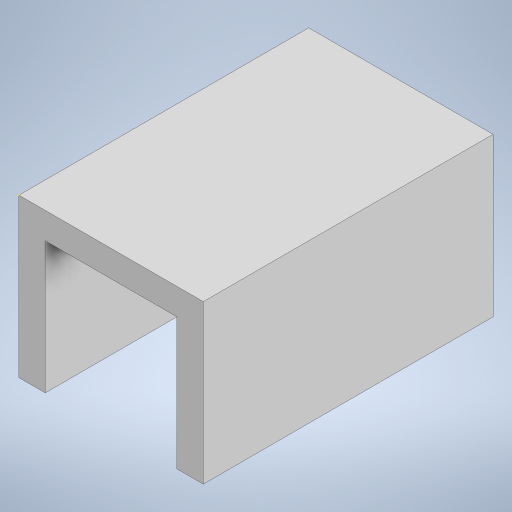
# Autodesk Inventor part: housing_v04
Saved by Autodesk Inventor 2023 (Build 270158000, 158)
## iProperties
Created: 2023-11-20
Part Number: housing_v04
Material: Generic
Document SubType Name: Modeling
Designer: Akramilab
Density: 1 g/cm^3
Appearance: Default
Author: Akramilab
Autodesk Inventor part; units mm, degrees
ref_plane "YZ Plane" through (0, 0, 0) normal (1, 0, 0) x (0, 1, 0)
ref_plane "XZ Plane" through (0, 0, 0) normal (0, 1, 0) x (-1, 0, 0)
ref_plane "XY Plane" through (0, 0, 0) normal (0, 0, 1) x (1, 0, 0)
sketch "Sketch1" plane through (0, 0, 0) normal (0, 0, 1) x (1, 0, 0)
  line L0 (0, 0) -> (14, 0)
  line L1 (14, 0) -> (14, -12)
  line L2 (14, -12) -> (0, -12)
  line L3 (0, -12) -> (0, 0)
  dimension "d0" = 14
  dimension "d1" = 12
  constraints: 8 end point, 2 parallel, 1 horizontal, 1 perpendicular
  measures "d0" distance of L1.end L2.end
  measures "d1" distance of L0.end L1.end
extrude "Extrusion1" add sketch "Sketch1" against normal blind 22
sketch "Sketch2" plane through (0, 0, 0) normal (0, 0, 1) x (1, 0, 0)
  line L0 (2, -2) -> (12, -2)
  line L1 (12, -2) -> (12, -22)
  line L2 (12, -22) -> (2, -22)
  line L3 (2, -22) -> (2, -2)
  point P0 (0, 0)
  dimension "d4" = 10
  dimension "d5" = 20
  constraints: 8 end point, 2 parallel, 1 horizontal, 1 perpendicular
  measures "d4" distance of L1.end L2.end
  measures "d5" distance of L0.end L1.end
extrude "Extrusion2" cut sketch "Sketch2" against normal blind 20
sketch "Sketch8" plane through (0, -12, 0) normal (-1, 0, 0) x (0, 0, 1)
  point P0 (0, 12)
sketch "Sketch9" plane through (0, -12, 0) normal (-1, 0, 0) x (0, 0, 1)
  point P0 (0, 12)
sketch "Sketch11" plane through (0, -12, 0) normal (-1, 0, 0) x (0, 0, 1)
  point P0 (0, 12)
sketch "Sketch12" plane through (0, -12, 0) normal (-1, 0, 0) x (0, 0, 1)
  line L0 (-11.5, 10) -> (-15.5, 10)
  line L1 (-15.5, 10) -> (-15.5, -1.8066)
  line L2 (-15.5, -1.8066) -> (-11.5, -1.8066)
  line L3 (-11.5, -1.8066) -> (-11.5, 10)
  point P0 (0, 12)
  dimension "d24" = 4
  constraints: 8 end point, 2 parallel, 1 horizontal, 1 perpendicular
  measures "d24" distance of L2.end L1.end
extrude "Extrusion8" cut sketch "Sketch12" against normal blind 10
body "Solid1"
